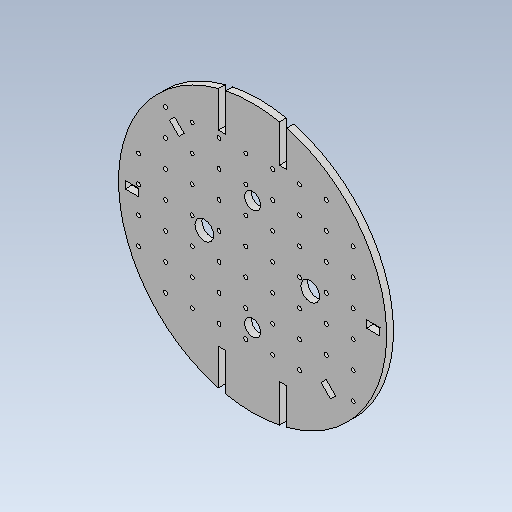
# Autodesk Inventor part: baseplate
Saved by Autodesk Inventor 2025 (Build 290162000, 162)
## iProperties
Created: 2024-08-12
Part Number: baseplate
Material: Polycarbonate, Clear
Document SubType Name: Modeling
Designer: PC
Density: 1.2 g/cm^3
Appearance: Default
Author: PC
Autodesk Inventor part; units mm, degrees
ref_plane "YZ Plane" through (0, 0, 0) normal (1, 0, 0) x (0, 1, 0)
ref_plane "XZ Plane" through (0, 0, 0) normal (0, 1, 0) x (-1, 0, 0)
ref_plane "XY Plane" through (0, 0, 0) normal (0, 0, 1) x (1, 0, 0)
sketch "Sketch2" plane through (0, 0, 0) normal (0, 0, 1) x (1, 0, 0)
  circle A0 centre (0, 0) radius 100
  line L0 (65, -65) -> (-65, -65) construction
  line L1 (-65, -65) -> (-65, 65) construction
  line L2 (-65, 65) -> (65, 65) construction
  line L3 (65, 65) -> (65, -65) construction
  line L4 (65, -65) -> (-65, 65) construction
  line L5 (-65, -65) -> (65, 65) construction
  line L6 (45, 45) -> (-45, 45) construction
  line L7 (-45, 45) -> (-45, -45) construction
  line L8 (-45, -45) -> (45, -45) construction
  line L9 (45, -45) -> (45, 45) construction
  line L10 (-25, 25) -> (25, 25) construction
  line L11 (25, 25) -> (25, -25) construction
  line L12 (25, -25) -> (-25, -25) construction
  line L13 (-25, -25) -> (-25, 25) construction
  line L14 (5, 5) -> (-5, 5) construction
  line L15 (-5, 5) -> (-5, -5) construction
  line L16 (-5, -5) -> (5, -5) construction
  line L17 (5, -5) -> (5, 5) construction
  circle A1 centre (-65, 65) radius 1.5
  circle A2 centre (-45, 65) radius 1.5
  circle A3 centre (-25, 65) radius 1.5
  circle A4 centre (-5, 65) radius 1.5
  circle A5 centre (15, 65) radius 1.5
  circle A6 centre (35, 65) radius 1.5
  circle A7 centre (55, 65) radius 1.5
  circle A8 centre (-65, 45) radius 1.5
  circle A9 centre (-65, 25) radius 1.5
  circle A10 centre (-65, 5) radius 1.5
  circle A11 centre (-65, -15) radius 1.5
  circle A12 centre (-65, -35) radius 1.5
  circle A13 centre (-65, -55) radius 1.5
  circle A14 centre (-45, 45) radius 1.5
  circle A15 centre (-25, 45) radius 1.5
  circle A16 centre (-5, 45) radius 1.5
  circle A17 centre (15, 45) radius 1.5
  circle A18 centre (35, 45) radius 1.5
  circle A19 centre (55, 45) radius 1.5
  circle A20 centre (-45, 25) radius 1.5
  circle A21 centre (-25, 25) radius 1.5
  circle A22 centre (-5, 25) radius 1.5
  circle A23 centre (15, 25) radius 1.5
  circle A24 centre (35, 25) radius 1.5
  circle A25 centre (55, 25) radius 1.5
  circle A26 centre (75, 25) radius 1.5
  circle A27 centre (-45, 5) radius 1.5
  circle A28 centre (-25, 5) radius 1.5
  circle A29 centre (-5, 5) radius 1.5
  circle A30 centre (15, 5) radius 1.5
  circle A31 centre (35, 5) radius 1.5
  circle A32 centre (55, 5) radius 1.5
  circle A33 centre (75, 5) radius 1.5
  circle A34 centre (-85, 25) radius 1.5
  circle A35 centre (-85, 5) radius 1.5
  circle A36 centre (-85, -15) radius 1.5
  circle A37 centre (-45, -15) radius 1.5
  circle A38 centre (-25, -15) radius 1.5
  circle A39 centre (-5, -15) radius 1.5
  circle A40 centre (15, -15) radius 1.5
  circle A41 centre (35, -15) radius 1.5
  circle A42 centre (55, -15) radius 1.5
  circle A43 centre (75, -15) radius 1.5
  circle A44 centre (-85, -35) radius 1.5
  circle A45 centre (-45, -35) radius 1.5
  circle A46 centre (-25, -35) radius 1.5
  circle A47 centre (-5, -35) radius 1.5
  circle A48 centre (15, -35) radius 1.5
  circle A49 centre (35, -35) radius 1.5
  circle A50 centre (55, -35) radius 1.5
  circle A51 centre (75, -35) radius 1.5
  circle A52 centre (-45, -55) radius 1.5
  circle A53 centre (-25, -55) radius 1.5
  circle A54 centre (-5, -55) radius 1.5
  circle A55 centre (15, -55) radius 1.5
  circle A56 centre (35, -55) radius 1.5
  circle A57 centre (55, -55) radius 1.5
  circle A58 centre (75, -55) radius 1.5
  circle A59 centre (75, 45) radius 1.5
  line L18 (-25.5, 96.6941) -> (-25.5, 69.8633)
  line L19 (-20, 97.9796) -> (-20, 69.8633)
  line L20 (0, 0) -> (0, 137.1728) construction
  line L21 (20, 97.9796) -> (20, 69.8633)
  line L22 (25.5, 96.6941) -> (25.5, 69.8633)
  line L23 (-20, 69.8633) -> (-25.5, 69.8633)
  line L24 (25.5, 69.8633) -> (20, 69.8633)
  line L25 (0, 0) -> (86, 0) construction
  line L26 (-25.5, -96.6941) -> (-25.5, -69.8633)
  line L27 (-20, -97.9796) -> (-20, -69.8633)
  line L28 (20, -97.9796) -> (20, -69.8633)
  line L29 (25.5, -96.6941) -> (25.5, -69.8633)
  line L30 (-20, -69.8633) -> (-25.5, -69.8633)
  line L31 (25.5, -69.8633) -> (20, -69.8633)
  circle A60 centre (0, 37) radius 6
  circle A61 centre (0, -45) radius 6
  circle A62 centre (-36, 0) radius 7
  circle A63 centre (43, 0) radius 7
  point P0 (-20, 99.8633)
  point P1 (-25.5, 99.8633)
  point P2 (22.75, 69.8633)
  point P3 (-25, 0)
  point P4 (-25.5, -96.6941)
  point P5 (25.5, -96.6941)
  dimension "d66" = 200
  dimension "d67" = 130
  dimension "d68" = 130
  dimension "d69" = 20
  dimension "d70" = 20
  dimension "d71" = 20
  dimension "d72" = 3
  dimension "d75" = 20
  dimension "d82" = 20
  dimension "d89" = 20
  dimension "d96" = 20
  dimension "d103" = 20
  dimension "d110" = 20
  dimension "d117" = 20
  dimension "d124" = 20
  dimension "d131" = 20
  dimension "d138" = 20
  dimension "d145" = 20
  dimension "d152" = 20
  dimension "d159" = 20
  dimension "d164" = 5.5
  dimension "d165" = 20
  dimension "d166" = 40
  dimension "d167" = 5.5
  dimension "d168" = 30
  dimension "d169" = 30
  dimension "d170" = 69.8633
  dimension "d176" = 12
  dimension "d177" = 37
  dimension "d178" = 12
  dimension "d179" = 14
  dimension "d180" = 11
  dimension "d181" = 97.9796
  dimension "d182" = 14
  dimension "d183" = 43
  constraints: 64 centre point, 64 end point, 15 horizontal, 12 parallel, 8 symmetric about line, 6 midpoint, 4 perpendicular, 4 point on circle, 3 point on line, 3 vertical, 2 coincident, 2 horizontal alignment, 125 other
  measures "d66" diameter of A0
  measures "d67" distance of L1.end L2.end
  measures "d68" distance of L0.end L1.end
  measures "d69" distance between parallel lines of L2 L6
  measures "d70" distance between parallel lines of L6 L10
  measures "d71" distance between parallel lines of L10 L14
  measures "d72" diameter of A1
  measures "d75" distance of A1.centre A2.centre
  measures "d82" distance of A1.centre A8.centre
  measures "d89" distance of A8.centre A14.centre
  measures "d96" distance of A9.centre A20.centre
  measures "d103" distance of A10.centre A27.centre
  measures "d110" distance of A9.centre A34.centre
  measures "d117" distance of A10.centre A35.centre
  measures "d124" distance of A11.centre A36.centre
  measures "d131" distance of A11.centre A37.centre
  measures "d138" distance of A12.centre A44.centre
  measures "d145" distance of A12.centre A45.centre
  measures "d152" distance of A13.centre A52.centre
  measures "d159" distance of A19.centre A59.centre
  measures "d164" distance between parallel lines of L18 L19
  measures "d165" distance between parallel lines of L20 L19
  measures "d166" distance between parallel lines of L19 L21
  measures "d167" distance between parallel lines of L21 L22
  measures "d168" distance of point (-20, 99.863) L19.end
  measures "d169" distance of point (-25.5, 99.863) L18.end
  measures "d170" vertical distance of L20.start point (22.75, 69.863)
  measures "d176" diameter of A60
  measures "d177" distance of point (0, 0) A60.centre
  measures "d178" diameter of A61
  measures "d179" diameter of A62
  measures "d180" distance of point (-25, 0) A62.centre
  measures "d181" vertical distance of L27.start A62.centre
  measures "d182" diameter of A63
  measures "d183" distance of point (0, 0) A63.centre
extrude "Extrusion1" add sketch "Sketch2" along normal blind 5.1 contours A0 L29 L31 L28 L27 L30 L26 L18 L23 L19 L21 L24 L22
sketch "Sketch3" plane through (0, 0, 5.1) normal (0, 0, 1) x (1, 0, 0)
  line L0 (-85, -2.92) -> (-95, -2.92)
  line L1 (-95, -2.92) -> (-95, 2.58)
  line L2 (-95, 2.58) -> (-85, 2.58)
  line L3 (-85, 2.58) -> (-85, -2.92)
  line L4 (-85, -2.92) -> (-95, 2.58) construction
  line L5 (-95, -2.92) -> (-85, 2.58) construction
  line L6 (0, 0) -> (0, -14.8693) construction
  line L7 (85, -2.92) -> (95, -2.92)
  line L8 (95, -2.92) -> (95, 2.58)
  line L9 (95, 2.58) -> (85, 2.58)
  line L10 (85, 2.58) -> (85, -2.92)
  line L11 (85, -2.92) -> (95, 2.58) construction
  line L12 (95, -2.92) -> (85, 2.58) construction
  point P0 (-90, -0.17)
  point P1 (-90, -2.92)
  point P2 (90, -0.17)
  point P3 (90, -2.92)
  dimension "d186" = 10
  dimension "d187" = 5.5
  dimension "d188" = 90
  constraints: 26 end point, 6 symmetric about line, 3 midpoint, 2 parallel, 1 horizontal, 1 perpendicular, 1 vertical
  measures "d186" distance of L1.end L2.end
  measures "d187" distance of L0.end L1.end
  measures "d188" horizontal distance of L6.start point (-90, -2.92)
extrude "Extrusion2" cut sketch "Sketch3" against normal blind 10
sketch "Sketch4" plane through (0, 0, 5.1) normal (0, 0, 1) x (1, 0, 0)
  line L0 (0, 0) -> (-90.4927, 90.4927) construction
  line L1 (0, 0) -> (-18.6759, 0) construction
  line L2 (0, 0) -> (-18.7177, -18.7177) construction
  line L3 (-85, -2.92) -> (-95, -2.92) projected
  line L4 (-95, 2.58) -> (-85, 2.58) projected
  line L5 (-85, 2.58) -> (-85, -2.92) projected
  line L6 (-62.0152, 58.1261) -> (-54.9441, 51.055)
  line L7 (-58.1261, 62.0152) -> (-51.055, 54.9441)
  line L8 (-58.1261, 62.0152) -> (-62.0152, 58.1261)
  line L9 (-51.055, 54.9441) -> (-54.9441, 51.055)
  line L10 (0, 0) -> (90.4927, -90.4927) construction
  line L11 (58.1261, -62.0152) -> (51.055, -54.9441)
  line L12 (62.0152, -58.1261) -> (54.9441, -51.055)
  line L13 (62.0152, -58.1261) -> (58.1261, -62.0152)
  line L14 (54.9441, -51.055) -> (51.055, -54.9441)
  point P0 (-58.4797, 54.5906)
  point P1 (-54.5906, 58.4797)
  point P2 (54.5906, -58.4797)
  point P3 (58.4797, -54.5906)
  dimension "d192" = 45
  dimension "d193" = 45
  dimension "d194" = 10
  dimension "d195" = 80
  dimension "d196" = 80
  dimension "d197" = 2.75
  dimension "d198" = 2.75
  constraints: 24 end point, 7 symmetric about line, 4 parallel, 2 midpoint, 1 horizontal
  measures "d192" angle of L1 L0
  measures "d193" angle of L2 L1
  measures "d194" distance of L6.start L6.end
  measures "d195" distance of L0.start point (-58.48, 54.591)
  measures "d196" distance of L0.start point (-54.591, 58.48)
  measures "d197" distance from line of L0 point (-54.591, 58.48)
  measures "d198" distance from line of L0 point (-58.48, 54.591)
extrude "Extrusion3" cut sketch "Sketch4" against normal blind 10
body "Solid1"
